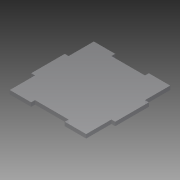
# Autodesk Inventor part: inside_box_left_right
Saved by Autodesk Inventor 2013 (Build 170138000, 138)
## iProperties
Created: 2014-05-23
Part Number: inside_box_left_right
Material: Polycarbonate, Clear
Document SubType Name: Modeling
Designer: balogh
Density: 1.2 g/cm^3
Mass: 12.7331 g
Surface Area: 80.9804 cm^2
Volume: 10.611 cm^3
Author: balogh
Autodesk Inventor part; units mm, degrees
ref_plane "YZ Plane" through (0, 0, 0) normal (1, 0, 0) x (0, 1, 0)
ref_plane "XZ Plane" through (0, 0, 0) normal (0, 1, 0) x (-1, 0, 0)
ref_plane "XY Plane" through (0, 0, 0) normal (0, 0, 1) x (1, 0, 0)
sketch "Sketch1" plane through (0, 0, 0) normal (0, 0, 1) x (1, 0, 0)
  line L0 (-12.7, 28.8544) -> (-28.8544, 28.8544)
  line L1 (-28.8544, 28.8544) -> (-31.75, 28.8544)
  line L2 (-31.75, 28.8544) -> (-31.75, 12.7)
  line L3 (-31.75, 12.7) -> (-28.8544, 12.7)
  line L4 (-28.8544, 12.7) -> (-28.8544, -12.7)
  line L5 (-28.8544, -12.7) -> (-31.75, -12.7)
  line L6 (-31.75, -12.7) -> (-31.75, -28.8544)
  line L7 (-31.75, -28.8544) -> (-28.8544, -28.8544)
  line L8 (-28.8544, -28.8544) -> (-12.7, -28.8544)
  line L9 (-12.7, -28.8544) -> (-12.7, -31.75)
  line L10 (-12.7, -31.75) -> (12.7, -31.75)
  line L11 (12.7, -31.75) -> (12.7, -28.8544)
  line L12 (12.7, -28.8544) -> (28.8544, -28.8544)
  line L13 (28.8544, -28.8544) -> (31.75, -28.8544)
  line L14 (31.75, -28.8544) -> (31.75, -12.7)
  line L15 (31.75, -12.7) -> (28.8544, -12.7)
  line L16 (28.8544, -12.7) -> (28.8544, 12.7)
  line L17 (28.8544, 12.7) -> (31.75, 12.7)
  line L18 (31.75, 12.7) -> (31.75, 28.8544)
  line L19 (31.75, 28.8544) -> (28.8544, 28.8544)
  line L20 (28.8544, 28.8544) -> (12.7, 28.8544)
  line L21 (12.7, 28.8544) -> (12.7, 31.75)
  line L22 (12.7, 31.75) -> (-12.7, 31.75)
  line L23 (-12.7, 31.75) -> (-12.7, 28.8544)
  point P0 (0, 0)
  constraints: 48 end point, 12 parallel, 6 perpendicular, 5 collinear
extrude "Extrusion1" add sketch "Sketch1" along normal blind 2.8956
body "Solid1"
